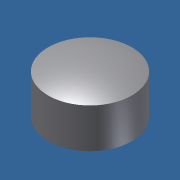
# Autodesk Inventor part: door knob
Saved by Autodesk Inventor 2012 (Build 160160000, 160)
## iProperties
Created: 2012-07-09
Part Number: door knob
Material: Default
Document SubType Name: Modeling
Designer: Ed
Density: 1 g/cm^3
Author: Ed
Autodesk Inventor part; units mm, degrees
ref_plane "YZ Plane" through (0, 0, 0) normal (1, 0, 0) x (0, 1, 0)
ref_plane "XZ Plane" through (0, 0, 0) normal (0, 1, 0) x (-1, 0, 0)
ref_plane "XY Plane" through (0, 0, 0) normal (0, 0, 1) x (1, 0, 0)
sketch "Sketch1" plane through (0, 0, 0) normal (0, 0, 1) x (1, 0, 0)
  arc A0 (28.6366, 34.8787) -> (0.1366, 39.8787) centre (0.1366, -43.8463) ccw
  line L0 (28.6366, 34.8787) -> (28.6366, 7.8787)
  line L1 (28.6366, 7.8787) -> (0.1366, 7.8787)
  line L2 (0.1366, 7.8787) -> (0.1366, 39.8787)
  point P0 (0, 0)
  point P1 (0.1366, 21.9958)
  dimension "d0" = 28.5
  dimension "d1" = 32
  dimension "d2" = 5
  constraints: 6 end point, 2 perpendicular, 2 point on circle, 2 vertical alignment, 1 centre point, 1 point on line, 1 vertical
  measures "d0" distance between parallel lines of L2 L0
  measures "d1" distance from line of L1 L2.end
  measures "d2" vertical distance of L2.end L0.start
revolve "Revolution1" add sketch "Sketch1" angle 360 about axis through (0.1366, 7.8787, 0) along (0, 1, 0)
body "Solid1"
